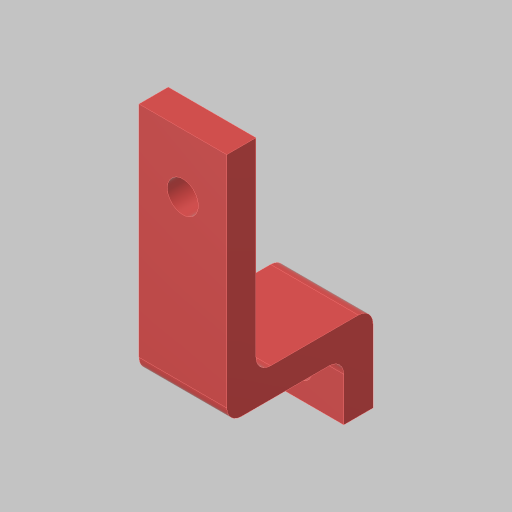
# Autodesk Inventor part: EL2-030
Saved by Autodesk Inventor 2023.5 (Build 275446000, 446)
## iProperties
Created: 2025-02-13
Part Number: EL2-030
Material: ABS Plastic
Document SubType Name: Modeling
Designer: slick
Density: 1.06 g/cm^3
Appearance: Smooth - Red
Author: slick
Autodesk Inventor part; units mm, degrees
ref_plane "YZ Plane" through (0, 0, 0) normal (1, 0, 0) x (0, 1, 0)
ref_plane "XZ Plane" through (0, 0, 0) normal (0, 1, 0) x (-1, 0, 0)
ref_plane "XY Plane" through (0, 0, 0) normal (0, 0, 1) x (1, 0, 0)
sketch "Sketch1" plane through (0, 0, 0) normal (1, 0, 0) x (0, 1, 0)
  line L0 (0, 0) -> (50.8, 0)
  line L1 (0, 0) -> (0, -25.4)
  line L2 (0, -25.4) -> (-12.7, -25.4)
  line L3 (50.8, -6.35) -> (6.35, -6.35)
  line L4 (6.35, -6.35) -> (6.35, -31.75)
  line L5 (6.35, -31.75) -> (-12.7, -31.75)
  line L6 (50.8, 0) -> (50.8, -6.35)
  line L7 (-12.7, -25.4) -> (-12.7, -31.75)
  dimension "d0" = 50.8
  dimension "d1" = 25.4
  dimension "d2" = 12.7
  dimension "d3" = 6.35
  constraints: 16 end point, 2 perpendicular, 2 vertical, 1 horizontal, 1 parallel, 2 other
  measures "d0" distance of L0.start L0.end
  measures "d1" distance of L0.start L1.end
  measures "d2" distance of L1.end L2.end
  measures "d3" distance between parallel lines of L0 L3
extrude "Extrusion1" add sketch "Sketch1" along normal blind 19.05
sketch "Sketch2" plane through (0, 0, 0) normal (0, 0, 1) x (1, 0, 0)
  line L0 (0, 50.8) -> (19.05, 50.8) construction
  line L1 (19.05, 6.35) -> (19.05, 50.8) construction
  point P0 (0, 0)
  point P1 (9.525, 38.1)
  point P2 (9.525, 50.8)
  point P3 (19.05, 28.575)
  dimension "d21" = 12.7
  constraints: 2 midpoint, 1 vertical alignment
  measures "d21" distance from line of L0 point (9.525, 38.1)
hole "Hole1" at (9.525, 38.1, 0) direction (0, 0, -1) diameter 6.7564 end through all clearance for "Flat Head Machine Screw (82)" size "1/4" standard "Ansi Unified Screw Threads"
sketch "Sketch3" plane through (0, -12.7, -25.4) normal (0, 0, 1) x (1, 0, 0)
  line L0 (0, 12.7) -> (0, 0) construction
  line L1 (0, 0) -> (19.05, 0) construction
  point P0 (9.525, 6.35)
  point P1 (0, 6.35)
  point P2 (9.525, 0)
  constraints: 2 midpoint, 1 horizontal alignment, 1 vertical alignment
hole "Hole2" at (9.525, -6.35, -25.4) direction (0, 0, -1) diameter 5.1054 end through all clearance for "Flat Head Machine Screw (82)" size "#10" standard "Ansi Unified Screw Threads"
fillet "Fillet1" radius 3.175 4 edges at (9.525, 6.35, -6.35) (9.525, 0, -25.4) (9.525, 6.35, -31.75) (9.525, 0, 0)
body "Solid1"
